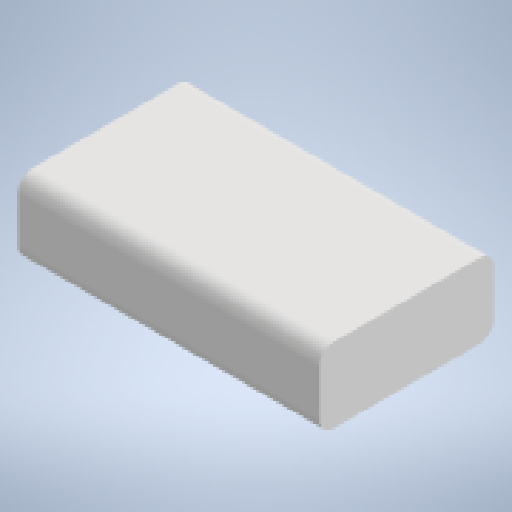
# Autodesk Inventor part: Battery box
Saved by Autodesk Inventor 2024 (Build 280153000, 153)
## iProperties
Created: 2024-09-18
Part Number: Battery box
Material: Generic
Document SubType Name: Modeling
Designer: NDurn
Density: 1 g/cm^3
Appearance: Default
Author: NDurn
Autodesk Inventor part; units mm, degrees
ref_plane "YZ Plane" through (0, 0, 0) normal (1, 0, 0) x (0, 1, 0)
ref_plane "XZ Plane" through (0, 0, 0) normal (0, 1, 0) x (-1, 0, 0)
ref_plane "XY Plane" through (0, 0, 0) normal (0, 0, 1) x (1, 0, 0)
sketch "Sketch1" plane through (0, 0, 0) normal (0, 1, 0) x (-1, 0, 0)
  line L0 (9.6242, 8.0407) -> (-53.8758, 8.0407)
  line L1 (-53.8758, 8.0407) -> (-53.8758, -28.7893)
  line L2 (-53.8758, -28.7893) -> (9.6242, -28.7893)
  line L3 (9.6242, -28.7893) -> (9.6242, 8.0407)
  point P0 (0, 0)
  dimension "d0" = 63.5
  dimension "d1" = 36.83
  constraints: 8 end point, 2 parallel, 1 horizontal, 1 perpendicular
  measures "d0" distance of L2.end L1.end
  measures "d1" distance of L1.end L0.end
extrude "Extrusion1" add sketch "Sketch1" along normal blind 15.748
fillet "Fillet1" radius 3.175 4 edges at (22.1258, 15.748, 8.0407) (22.1258, 15.748, -28.7893) (22.1258, 0, 8.0407) (22.1258, 0, -28.7893)
body "Solid1"
